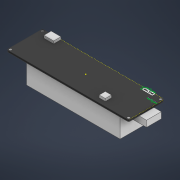
# Autodesk Inventor part: battery_footprint
Saved by Autodesk Inventor 2021 (Build 250183000, 183)
## iProperties
Created: 2021-12-18
Part Number: battery_footprint
Material: Generic
Document SubType Name: Modeling
Designer: Juan M. Casillas
Density: 1 g/cm^3
Appearance: Default
Author: Juan M. Casillas
Autodesk Inventor part; units mm, degrees
ref_plane "YZ Plane" through (0, 0, 0) normal (1, 0, 0) x (0, 1, 0)
ref_plane "XZ Plane" through (0, 0, 0) normal (0, 1, 0) x (-1, 0, 0)
ref_plane "XY Plane" through (0, 0, 0) normal (0, 0, 1) x (1, 0, 0)
sketch "Sketch1" plane through (0, 0, 0) normal (0, 1, 0) x (-1, 0, 0)
  line L0 (49.5, 14.5) -> (-49.5, 14.5)
  line L1 (-49.5, 14.5) -> (-49.5, -14.5)
  line L2 (-49.5, -14.5) -> (49.5, -14.5)
  line L3 (49.5, -14.5) -> (49.5, 14.5)
  line L4 (49.5, 14.5) -> (-49.5, -14.5) construction
  line L5 (-49.5, 14.5) -> (49.5, -14.5) construction
  point P0 (0, 0)
  dimension "d0" = 99
  dimension "d1" = 29
  constraints: 12 end point, 2 midpoint, 2 parallel, 1 horizontal, 1 perpendicular
  measures "d0" distance of L2.end L1.end
  measures "d1" distance of L1.end L0.end
extrude "Extrusion1" add sketch "Sketch1" along normal blind 1.5
fillet "Fillet1" radius 1 4 edges at (49.5, 0.75, 14.5) (49.5, 0.75, -14.5) (-49.5, 0.75, -14.5) (-49.5, 0.75, 14.5)
sketch "Sketch2" plane through (0, 1.5, 0) normal (0, 1, 0) x (1, 0, 0)
  line L0 (26.9904, -10.9774) -> (21.9904, -10.9774)
  line L1 (21.9904, -10.9774) -> (21.9904, -5.9774)
  line L2 (21.9904, -5.9774) -> (26.9904, -5.9774)
  line L3 (26.9904, -5.9774) -> (26.9904, -10.9774)
  line L4 (26.9904, -10.9774) -> (21.9904, -5.9774) construction
  line L5 (21.9904, -10.9774) -> (26.9904, -5.9774) construction
  point P0 (0, 0)
  point P1 (24.4904, -8.4774)
  dimension "d5" = 5
  dimension "d6" = 5
  constraints: 12 end point, 2 midpoint, 2 parallel, 1 horizontal, 1 perpendicular
  measures "d5" distance of L1.end L2.end
  measures "d6" distance of L0.end L1.end
extrude "Extrusion2" add sketch "Sketch2" along normal blind 2
sketch "Sketch3" plane through (0, 1.5, 0) normal (0, 1, 0) x (1, 0, 0)
  line L0 (26.9904, -5.9774) -> (26.9904, -10.9774) construction
  line L1 (26.9904, -10.9774) -> (21.9904, -10.9774) construction
  line L2 (21.9904, -10.9774) -> (21.9904, -5.9774) construction
  line L3 (21.9904, -5.9774) -> (26.9904, -5.9774) construction
  arc A0 (-49.5, -13.5) -> (-48.5, -14.5) centre (-48.5, -13.5) ccw construction
  line L4 (-48.5, -14.5) -> (48.5, -14.5) construction
  arc A1 (48.5, -14.5) -> (49.5, -13.5) centre (48.5, -13.5) ccw construction
  line L5 (49.5, -13.5) -> (49.5, 13.5) construction
  arc A2 (49.5, 13.5) -> (48.5, 14.5) centre (48.5, 13.5) ccw construction
  line L6 (48.5, 14.5) -> (-48.5, 14.5) construction
  arc A3 (-48.5, 14.5) -> (-49.5, 13.5) centre (-48.5, 13.5) ccw construction
  line L7 (-49.5, 13.5) -> (-49.5, -13.5) construction
  line L8 (48, -13) -> (-48, -13) construction
  line L9 (-48, -13) -> (-48, 13) construction
  line L10 (-48, 13) -> (48, 13) construction
  line L11 (48, 13) -> (48, -13) construction
  point P0 (0, 0)
  dimension "d9" = 1.5
  constraints: 8 end point, 4 coincident, 3 other
  measures "d9" distance between parallel lines of L4 L8
hole "Hole1" at (48, 1.5, 13) at (-48, 1.5, 13) at (-48, 1.5, -13) at (48, 1.5, -13) direction (0, -1, 0) diameter 2 depth 10 tip angle 118
sketch "Sketch4" plane through (0, 1.5, 0) normal (0, 1, 0) x (1, 0, 0)
  line L0 (-49.5, 13.5) -> (-49.5, -13.5) construction
  line L1 (-49.5, 10.3219) -> (-42.5, 10.3219) construction
  line L2 (-34.5, 8.5) -> (-42.5, 8.5)
  line L3 (-42.5, 8.5) -> (-42.5, 14.5)
  line L4 (-42.5, 14.5) -> (-34.5, 14.5)
  line L5 (-34.5, 14.5) -> (-34.5, 8.5)
  line L6 (-34.5, 8.5) -> (-42.5, 14.5) construction
  line L7 (-42.5, 8.5) -> (-34.5, 14.5) construction
  line L8 (48.5, 14.5) -> (-48.5, 14.5) construction
  point P0 (0, 0)
  point P1 (-38.5, 11.5)
  dimension "d17" = 7
  dimension "d18" = 8
  dimension "d19" = 6
  constraints: 14 end point, 2 horizontal, 2 midpoint, 2 parallel, 2 point on line, 1 collinear, 1 perpendicular
  measures "d17" distance of L1.start L1.end
  measures "d18" distance of L3.end L4.end
  measures "d19" distance of L2.end L3.end
extrude "Extrusion3" add sketch "Sketch4" along normal blind 2
sketch "Sketch5" plane through (0, 1.5, 0) normal (0, 1, 0) x (1, 0, 0)
  line L0 (49.5, -13.5) -> (49.5, 13.5) construction
  line L1 (49.5, 9.2214) -> (41.5, 9.2214) construction
  line L2 (48.5, 14.5) -> (-34.5, 14.5) construction
  line L3 (41.5, 12.5) -> (33.5, 12.5)
  line L4 (33.5, 12.5) -> (33.5, 14.5)
  line L5 (33.5, 14.5) -> (41.5, 14.5)
  line L6 (41.5, 14.5) -> (41.5, 12.5)
  line L7 (41.5, 12.5) -> (33.5, 14.5) construction
  line L8 (33.5, 12.5) -> (41.5, 14.5) construction
  point P0 (0, 0)
  point P1 (37.5, 13.5)
  dimension "d22" = 8
  dimension "d23" = 8
  dimension "d24" = 2
  constraints: 14 end point, 2 midpoint, 2 parallel, 2 perpendicular, 2 point on line, 1 collinear, 1 horizontal
  measures "d22" distance of L1.start L1.end
  measures "d23" distance of L4.end L5.end
  measures "d24" distance of L3.end L4.end
sketch "Sketch6" plane through (0, 0, 0) normal (0, -1, 0) x (1, 0, 0)
  line L0 (41.5, -12.5) -> (33.5, -12.5) projected
  line L1 (41.5, -14.5) -> (41.5, -12.5) projected
  line L2 (33.5, -12.5) -> (33.5, -14.5) projected
  line L3 (41.5, -14.5) -> (33.5, -14.5)
  point P0 (0, 0)
  constraints: 2 end point, 1 horizontal
extrude "Extrusion4" add sketch "Sketch6" along normal blind 2
sketch "Sketch7" plane through (0, 0, 0) normal (0, -1, 0) x (1, 0, 0)
  line L0 (33.5, -14.5) -> (33.5, -12.5) construction
  line L1 (33.5, -12.5) -> (41.5, -12.5) construction
  line L2 (41.5, -12.5) -> (41.5, -14.5) construction
  line L3 (48.5, -14.5) -> (41.5, -14.5) construction
  arc A0 (48.5, -14.5) -> (49.5, -13.5) centre (48.5, -13.5) ccw construction
  line L4 (49.5, 13.5) -> (49.5, -13.5) construction
  arc A1 (49.5, 13.5) -> (48.5, 14.5) centre (48.5, 13.5) ccw construction
  line L5 (-48.5, 14.5) -> (48.5, 14.5) construction
  arc A2 (-48.5, 14.5) -> (-49.5, 13.5) centre (-48.5, 13.5) ccw construction
  line L6 (-49.5, -13.5) -> (-49.5, 13.5) construction
  arc A3 (-49.5, -13.5) -> (-48.5, -14.5) centre (-48.5, -13.5) ccw construction
  line L7 (33.5, -14.5) -> (-48.5, -14.5) construction
  circle A4 centre (48, -13) radius 1 construction
  circle A5 centre (-48, 13) radius 1 construction
  circle A6 centre (48, 13) radius 1 construction
  circle A7 centre (-48, -13) radius 1 construction
  line L8 (55.5, -6) -> (41.5, -6)
  line L9 (41.5, -6) -> (41.5, 6)
  line L10 (41.5, 6) -> (55.5, 6)
  line L11 (55.5, 6) -> (55.5, -6)
  line L12 (55.5, -6) -> (41.5, 6) construction
  line L13 (41.5, -6) -> (55.5, 6) construction
  line L14 (49.5, 0) -> (55.5, 0) construction
  point P0 (0, 0)
  point P1 (48.5, 0)
  dimension "d27" = 14
  dimension "d28" = 12
  dimension "d29" = 6
  constraints: 14 end point, 4 midpoint, 2 horizontal, 2 parallel, 1 perpendicular
  measures "d27" distance of L9.end L10.end
  measures "d28" distance of L8.end L9.end
  measures "d29" distance of L14.end L14.start
extrude "Extrusion5" add sketch "Sketch7" along normal blind 5
sketch "Sketch8" plane through (0, 0, 0) normal (0, -1, 0) x (1, 0, 0)
  line L0 (41.5, 6) -> (49.5, 6) construction
  line L1 (49.5, 13.5) -> (49.5, 6) construction
  arc A0 (49.5, 13.5) -> (48.5, 14.5) centre (48.5, 13.5) ccw construction
  line L2 (-48.5, 14.5) -> (48.5, 14.5) construction
  arc A1 (-48.5, 14.5) -> (-49.5, 13.5) centre (-48.5, 13.5) ccw construction
  line L3 (-49.5, -13.5) -> (-49.5, 13.5) construction
  arc A2 (-49.5, -13.5) -> (-48.5, -14.5) centre (-48.5, -13.5) ccw construction
  line L4 (33.5, -14.5) -> (-48.5, -14.5) construction
  line L5 (33.5, -14.5) -> (33.5, -12.5) construction
  line L6 (33.5, -12.5) -> (41.5, -12.5) construction
  line L7 (41.5, -12.5) -> (41.5, -14.5) construction
  line L8 (48.5, -14.5) -> (41.5, -14.5) construction
  arc A3 (48.5, -14.5) -> (49.5, -13.5) centre (48.5, -13.5) ccw construction
  line L9 (49.5, -6) -> (49.5, -13.5) construction
  line L10 (49.5, -6) -> (41.5, -6) construction
  line L11 (41.5, -6) -> (41.5, 6) construction
  circle A4 centre (48, -13) radius 1 construction
  circle A5 centre (-48, 13) radius 1 construction
  circle A6 centre (48, 13) radius 1 construction
  circle A7 centre (-48, -13) radius 1 construction
  line L12 (38, -10) -> (-38, -10)
  line L13 (-38, -10) -> (-38, 10)
  line L14 (-38, 10) -> (38, 10)
  line L15 (38, 10) -> (38, -10)
  line L16 (38, -10) -> (-38, 10) construction
  line L17 (-38, -10) -> (38, 10) construction
  point P0 (0, 0)
  point P1 (0, 0)
  point P2 (0, 0)
  dimension "d32" = 76
  dimension "d33" = 20
  constraints: 12 end point, 3 midpoint, 2 parallel, 1 coincident, 1 horizontal, 1 perpendicular
  measures "d32" distance of L13.end L14.end
  measures "d33" distance of L12.end L13.end
extrude "Extrusion6" add sketch "Sketch8" along normal blind 20
body "Solid1"
